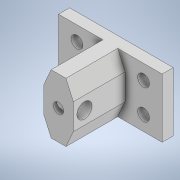
# Autodesk Inventor part: Guider
Saved by Autodesk Inventor 2021 (Build 250183000, 183)
## iProperties
Created: 2024-06-21
Part Number: Guider
Material: Generic
Document SubType Name: Modeling
Designer: Lukas
Density: 1 g/cm^3
Appearance: Default
Author: Lukas
Autodesk Inventor part; units mm, degrees
ref_plane "YZ Plane" through (0, 0, 0) normal (1, 0, 0) x (0, 1, 0)
ref_plane "XZ Plane" through (0, 0, 0) normal (0, 1, 0) x (-1, 0, 0)
ref_plane "XY Plane" through (0, 0, 0) normal (0, 0, 1) x (1, 0, 0)
sketch "Sketch1" plane through (0, 0, 0) normal (0, 0, 1) x (1, 0, 0)
  line L0 (-14, 8) -> (14, 8)
  line L1 (14, 8) -> (14, -8)
  line L2 (14, -8) -> (-14, -8)
  line L3 (-14, -8) -> (-14, 8)
  circle A0 centre (-9, 4) radius 1.6
  circle A1 centre (-9, -4) radius 1.6
  circle A2 centre (9, -4) radius 1.6
  circle A3 centre (9, 4) radius 1.6
  point P0 (0, 0)
  point P1 (0, 8)
  point P2 (-14, 0)
  dimension "d0" = 28
  dimension "d1" = 16
  dimension "d2" = 18
  dimension "d3" = 9
  dimension "d4" = 8
  dimension "d5" = 4
  dimension "d6" = 3.2
  constraints: 8 end point, 4 centre point, 3 equal radius, 3 horizontal alignment, 3 vertical alignment, 2 midpoint, 2 parallel, 1 horizontal, 1 perpendicular
  measures "d0" distance of L0.start L0.end
  measures "d1" distance of L0.end L1.end
  measures "d2" distance of A3.centre A0.centre
  measures "d3" horizontal distance of point (0, 0) A0.centre
  measures "d4" distance of A1.centre A0.centre
  measures "d5" vertical distance of point (0, 0) A0.centre
  measures "d6" diameter of A0
extrude "Extrusion1" add sketch "Sketch1" along normal blind 3
sketch "Sketch2" plane through (0, 0, 3) normal (0, 0, 1) x (1, 0, 0)
  line L0 (-4, -3.5) -> (-4, 3.5)
  line L1 (-4, 3.5) -> (-2, 8)
  line L2 (14, 8) -> (-14, 8) projected
  line L3 (-2, 8) -> (2, 8)
  line L4 (2, 8) -> (4, 3.5)
  line L5 (4, 3.5) -> (4, -3.5)
  line L6 (14, 8) -> (-14, 8) projected
  line L7 (4, -3.5) -> (2, -8)
  line L8 (-14, -8) -> (14, -8) projected
  line L9 (2, -8) -> (-2, -8)
  line L10 (-2, -8) -> (-4, -3.5)
  point P0 (0, 0)
  point P1 (-4, 0)
  point P2 (4, 0)
  point P3 (0, 8)
  dimension "d9" = 8
  dimension "d10" = 4
  dimension "d11" = 7
  constraints: 16 end point, 4 equal length, 4 point on line, 3 midpoint, 2 horizontal alignment, 1 perpendicular, 1 vertical, 1 vertical alignment
  measures "d9" distance between parallel lines of L5 L0
  measures "d10" distance of L3.end L1.end
  measures "d11" distance of L0.start L0.end
extrude "Extrusion2" add sketch "Sketch2" along normal blind 14
sketch "Sketch3" plane through (-4, -3.5, 3) normal (-1, 0, 0) x (0, 0, 1)
  circle A0 centre (11, 3.5) radius 2.05
  line L0 (14, 7) -> (14, 0) projected
  point P0 (-3, 3.5)
  point P1 (14, 3.5)
  dimension "d14" = 3
  dimension "d15" = 4.1
  constraints: 1 centre point, 1 horizontal alignment, 1 midpoint
  measures "d14" distance from line of L0 A0.centre
  measures "d15" diameter of A0
extrude "Extrusion3" cut sketch "Sketch3" against normal through all
sketch "Sketch4" plane through (0, 0, 17) normal (0, 0, 1) x (1, 0, 0)
  circle A0 centre (0, 0) radius 1.4
  dimension "d18" = 2.8
  constraints: 1 centre point, 1 coincident
  measures "d18" diameter of A0
extrude "Extrusion4" cut sketch "Sketch4" against normal blind 3
equation "\"d3\" = 0.5 * d2"
equation "\"d5\" = 0.5 * d4"
body "Solid1"
